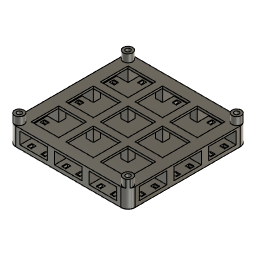
board_holder_outer_ziptie (Autodesk Fusion 360 design; units mm, degrees)
Autodesk Fusion 360 part; units mm, degrees
note: some values were not read from the file. Chosen so that the rebuilt part matches the saved one: which face or edge a step refers to.
sketch "Sketch1" plane through (0, 0, 0) normal (0, 0, 1) x (1, 0, 0)
  line L0 (-45.5, -45.5) -> (45.5, -45.5) construction
  line L1 (45.5, -45.5) -> (45.5, 45.5) construction
  line L2 (45.5, 45.5) -> (-45.5, 45.5) construction
  line L3 (-45.5, 45.5) -> (-45.5, -45.5) construction
  line L4 (-45.5, -45.5) -> (45.5, 45.5) construction
  line L5 (45.5, -45.5) -> (-45.5, 45.5) construction
  circle A0 centre (-45.5, 45.5) radius 1.95
  circle A1 centre (45.5, 45.5) radius 1.95
  circle A2 centre (-45.5, -45.5) radius 1.95
  circle A3 centre (45.5, -45.5) radius 1.95
  line L6 (-50, 50) -> (50, 50)
  line L7 (50, 50) -> (50, -50)
  line L8 (50, -50) -> (-50, -50)
  line L9 (-50, -50) -> (-50, 50)
  line L10 (-50, 50) -> (50, -50) construction
  line L11 (50, 50) -> (-50, -50) construction
  circle A4 centre (-45.5, 45.5) radius 3.95
  circle A5 centre (45.5, 45.5) radius 3.95
  circle A6 centre (-45.5, -45.5) radius 3.95
  circle A7 centre (45.5, -45.5) radius 3.95
  dimension "d1" = 91
  dimension "d2" = 91
  dimension "d3" = 3.9
  dimension "d6" = 91
  dimension "d8" = 100
  dimension "d9" = 7.9
  dimension "d12" = 91
  dimension "d102" = 100
  constraint perpendicular L0 L1
  constraint parallel L0 L2
  constraint parallel L1 L3
  constraint horizontal L0
  constraint coincident L4 origin
  constraint coincident L5 origin
  constraint coincident L2.end L3.start
  constraint perpendicular L6 L7
  constraint parallel L6 L8
  constraint parallel L7 L9
  constraint horizontal L6
  constraint coincident L10 origin
  constraint coincident L11 origin
  constraint concentric A0 A4
  measures "d1" distance of L1.end L2.end
  measures "d2" distance of L0.end L1.end
  measures "d3" diameter of A0
  measures "d8" distance of L7.end L8.end
  measures "d9" diameter of A4
  measures "d102" distance of L6.start L8.end
extrude "Extrude1" add sketch "Sketch1" along normal blind 18.5 contours A4 | A5 | A6 | A7 makes body 1 at (-41.5696, 45.1067, 6.1667) makes body 2 at (49.4304, 45.1067, 6.1667) makes body 3 at (-41.5696, -45.8933, 6.1667) makes body 4 at (49.4304, -45.8933, 6.1667)
extrude "Extrude2" add sketch "Sketch1" against normal blind 3.5 contours L6 L7 L8 L9 | A4 | A5 | A6 | A7 bodies 1 2 3 4
extrude "Extrude3" add sketch "Sketch1" along normal blind 12 contours L6 L7 L8 L9 bodies 1
sketch "Sketch2" plane through (0, -50, 0) normal (0, -1, 0) x (1, 0, 0)
  line L0 (50, -3.5) -> (50, 12)
  line L1 (-50, 12) -> (-40.5, 12)
  line L2 (-40.5, 12) -> (-40.5, -3.5)
  line L3 (-40.5, -3.5) -> (-50, -3.5)
  line L4 (-50, -3.5) -> (-50, 12)
  line L5 (-40.5, 12) -> (-17.5, 12)
  line L6 (-17.5, 12) -> (-17.5, -3.5)
  line L7 (-17.5, -3.5) -> (-40.5, -3.5)
  line L8 (-40.5, -3.5) -> (-40.5, 12)
  line L9 (-50, 12) -> (-50, 10)
  line L10 (-50, -3.5) -> (-50, 0)
  line L11 (-50, 10) -> (50, 10)
  line L12 (-50, 0) -> (50, 0)
  point P0 (-50, 12)
  dimension "d64" = 15.5
  dimension "d65" = 9.5
  dimension "d66" = 15.5
  dimension "d67" = 23
  dimension "d68" = 2
  dimension "d69" = 3.5
  constraint horizontal L1
  constraint vertical L2
  constraint horizontal L3
  constraint vertical L4
  constraint horizontal L5
  constraint vertical L6
  constraint horizontal L7
  constraint vertical L8
  constraint perpendicular L1 L9
  constraint perpendicular L3 L10
  constraint coincident L0 L11.end
  constraint perpendicular L0 L11
  constraint coincident L0 L12.end
  constraint perpendicular L0 L12
  constraint coincident P0 L1.start
  measures "d64" distance of P0 L3.end
  measures "d65" distance of P0 L1.end
  measures "d66" distance of L1.end L2.end
  measures "d67" distance of L1.end L5.end
  measures "d68" distance of P0 L9.end
  measures "d69" distance of L3.end L10.end
sketch "Sketch3" plane through (50, 0, 0) normal (1, 0, 0) x (0, 1, 0)
  line L0 (-50, 12) -> (-50, -3.5)
  line L1 (-50, -3.5) -> (50, -3.5)
  line L2 (50, -3.5) -> (50, 12)
  line L3 (50, 12) -> (-50, 12)
  line L4 (-50, 12) -> (-40.5, 12)
  line L5 (-40.5, 12) -> (-40.5, -3.5)
  line L6 (-40.5, -3.5) -> (-50, -3.5)
  line L7 (-50, -3.5) -> (-50, 12)
  line L8 (-40.5, 12) -> (-17.5, 12)
  line L9 (-17.5, 12) -> (-17.5, -3.5)
  line L10 (-17.5, -3.5) -> (-40.5, -3.5)
  line L11 (-40.5, -3.5) -> (-40.5, 12)
  line L12 (-50, 12) -> (-50, 10.3)
  line L13 (-50, -3.5) -> (-50, 0)
  line L14 (-50, 10.3) -> (50, 10.3)
  line L15 (-50, 0) -> (50, 0)
  dimension "d85" = 9.5
  dimension "d86" = 15.5
  dimension "d87" = 23
  dimension "d88" = 15.5
  dimension "d89" = 1.7
  dimension "d90" = 3.5
  constraint horizontal L4
  constraint vertical L5
  constraint horizontal L6
  constraint vertical L7
  constraint coincident L0.start L3.end
  constraint horizontal L8
  constraint vertical L9
  constraint horizontal L10
  constraint vertical L11
  constraint perpendicular L3 L12
  constraint coincident L0.end L1.start
  constraint perpendicular L6 L13
  constraint coincident L2 L14.end
  constraint perpendicular L2 L14
  constraint coincident L2 L15.end
  constraint perpendicular L2 L15
  measures "d85" distance of L0.start L4.end
  measures "d86" distance of L0.start L0.end
  measures "d87" distance of L4.end L8.end
  measures "d88" distance of L4.end L5.end
  measures "d89" distance of L0.start L12.end
  measures "d90" distance of L0.end L13.end
sketch "Sketch4" plane through (0, 0, -3.5) normal (0, 0, -1) x (1, 0, 0)
  circle A0 centre (-45.5, 45.5) radius 1.95
  circle A1 centre (45.5, 45.5) radius 1.95
  line L0 (50, 50) -> (-50, 50)
  line L1 (-50, 50) -> (-50, -50)
  line L2 (-50, -50) -> (50, -50)
  line L3 (50, -50) -> (50, 50)
  line L4 (45.5, 45.5) -> (18.5, 45.5)
  line L5 (18.5, 45.5) -> (18.5, 18.5)
  line L6 (18.5, 18.5) -> (45.5, 18.5)
  line L7 (45.5, 18.5) -> (45.5, 45.5)
  circle A2 centre (18.5, 18.5) radius 6.5
  circle A3 centre (-45.5, -45.5) radius 1.95
  circle A4 centre (45.5, -45.5) radius 1.95
  dimension "d43" = 27
  dimension "d44" = 27
  dimension "d45" = 13
  constraint horizontal L4
  constraint vertical L5
  constraint horizontal L6
  constraint vertical L7
  constraint coincident A1.centre L4.start
  constraint coincident L5.end L6.start
  measures "d43" distance of A1.centre L4.end
  measures "d44" distance of A1.centre L6.end
  measures "d45" diameter of A2
extrude "Extrude10" cut sketch "Sketch3" against normal blind 100 contours L5 L9 L11 L14 L15 bodies 1
pattern_linear "R-Pattern2" count 3 spacing 29 along (0, 1, 0) of "Extrude10"
extrude "Extrude9" cut sketch "Sketch2" against normal blind 100 contours L2 L6 L8 L11 L12 bodies 1
pattern_linear "R-Pattern1" count 3 spacing 29 along (1, 0, 0) of "Extrude9"
ref_plane "WorkPlane1" through (0, 0, 12) normal (0, 0, 1) x (1, 0, 0)
sketch "Sketch6" plane through (0, 0, 12) normal (0, 0, 1) x (1, 0, 0)
  line L0 (-50, 50) -> (50, 50) construction
  line L1 (50, 50) -> (50, -50) construction
  line L2 (50, -50) -> (-50, -50) construction
  line L3 (-50, -50) -> (-50, 50) construction
  line L4 (-50, 50) -> (50, -50) construction
  line L5 (50, 50) -> (-50, -50) construction
  line L6 (-50, -50) -> (-40.5, -50) construction
  line L7 (-40.5, -50) -> (-40.5, -40.5) construction
  line L8 (-40.5, -40.5) -> (-50, -40.5) construction
  line L9 (-50, -40.5) -> (-50, -50) construction
  line L10 (-40.5, -40.5) -> (-17.5, -40.5)
  line L11 (-17.5, -40.5) -> (-17.5, -17.5)
  line L12 (-17.5, -17.5) -> (-40.5, -17.5)
  line L13 (-40.5, -17.5) -> (-40.5, -40.5)
  dimension "d106" = 100
  dimension "d107" = 100
  dimension "d108" = 9.5
  dimension "d109" = 9.5
  dimension "d110" = 23
  dimension "d111" = 23
  constraint perpendicular L0 L1
  constraint parallel L0 L2
  constraint parallel L1 L3
  constraint horizontal L0
  constraint coincident L4 origin
  constraint coincident L5 origin
  constraint horizontal L6
  constraint vertical L7
  constraint horizontal L8
  constraint vertical L9
  constraint horizontal L10
  constraint vertical L11
  constraint horizontal L12
  constraint vertical L13
  measures "d106" distance of L1.end L2.end
  measures "d107" distance of L0.end L1.end
  measures "d108" distance of L2.end L6.end
  measures "d109" distance of L2.end L8.end
  measures "d110" distance of L7.end L10.end
  measures "d111" distance of L7.end L12.end
extrude "Extrude11" cut sketch "Sketch6" against normal blind 2 bodies 1
pattern_linear "R-Pattern3" count 3 spacing 29 along (0, 1, 0) count 3 spacing 29 along (1, 0, 0) of "Extrude11"
fillet "Fillet1" radius 6 4 edges at (-50, -50, 4.25) (50, -50, 4.25) (50, 50, 4.25) (-50, 50, 4.25) on bodies 1
chamfer "Chamfer3" distance 0.4 angle 45 12 edges at (-47.318, -46.2052, -3.5) (43.682, -46.2052, -3.5) (43.682, 44.7948, -3.5) (-47.318, 44.7948, -3.5) (0, 50, -3.5) (-48.2426, 48.2426, -3.5) (-50, 0, -3.5) (-48.2426, -48.2426, -3.5) (0, -50, -3.5) (48.2426, -48.2426, -3.5) (50, 0, -3.5) (48.2426, 48.2426, -3.5) on bodies 1
ref_plane "WorkPlane2" through (0, -46, 0) normal (0, 1, 0) x (0, 0, 1)
sketch "Sketch7" plane through (0, -46, 0) normal (0, 1, 0) x (1, 0, 0)
  line L0 (0, 0) -> (-50, 0) construction
  line L1 (-50, 0) -> (-40.5, 0) construction
  line L2 (-40.5, 0) -> (-29, 0) construction
  line L3 (-29, 0) -> (-29, 3.5) construction
  line L4 (-29, 0) -> (-27.625, 0) construction
  line L5 (-29, 0) -> (-33, 0) construction
  line L6 (-29, 3.5) -> (-40.5, 3.5) construction
  line L7 (-33, 0) -> (-33, 1)
  line L8 (-33, 0) -> (-35.5, 0)
  line L9 (-35.5, 0) -> (-35.5, 1)
  arc A0 (-33, 3.5) -> (-35.5, 1) centre (-33, 1) ccw
  line L10 (-33, 1) -> (-29, 1)
  line L11 (-33, 3.5) -> (-29, 3.5)
  line L12 (-29, 3.5) -> (-29, 1)
  arc A1 (-22.5, 1) -> (-25, 3.5) centre (-25, 1) ccw
  line L13 (-25, 0) -> (-22.5, 0)
  line L14 (-22.5, 0) -> (-22.5, 1)
  line L15 (-25, 0) -> (-25, 1)
  line L16 (-25, 1) -> (-29, 1)
  line L17 (-29, 3.5) -> (-17.5, 3.5) construction
  line L18 (-25, 3.5) -> (-29, 3.5)
  dimension "d121" = 50
  dimension "d122" = 9.5
  dimension "d123" = 11.5
  dimension "d124" = 3.5
  dimension "d126" = 4
  dimension "d127" = 11.5
  dimension "d128" = 1
  dimension "d129" = 2.5
  dimension "d130" = 1
  constraint coincident L0.start origin
  constraint horizontal L0
  constraint parallel L0 L1
  constraint parallel L0 L2
  constraint perpendicular L2 L3
  constraint perpendicular L3 L4
  constraint perpendicular L3 L5
  constraint perpendicular L3 L6
  constraint perpendicular L5 L7
  constraint perpendicular L7 L8
  constraint perpendicular L0 L9
  constraint coincident L6 A0.start
  constraint coincident L7.end A0.centre
  constraint coincident L3 L10.end
  constraint perpendicular L3 L10
  constraint symmetric L3.end L12 L6.start
  constraint symmetric L5.end L12 L13.start
  constraint symmetric L6.end L12 L17.end
  constraint symmetric L7.end L12 A1.centre
  constraint symmetric L8.end L12 L13.end
  constraint symmetric L9.end L12 A1.start
  constraint symmetric A0.start L12 A1.end
  constraint symmetric A0 L12 A1
  constraint symmetric L10.end L12 L16.end
  measures "d121" distance of L0.start L0.end
  measures "d122" distance of L0.end L1.end
  measures "d123" distance of L1.end L2.end
  measures "d124" distance of L2.end L3.end
  measures "d126" distance of L2.end L5.end
  measures "d127" distance of L3.end L6.end
  measures "d128" distance of L5.end L7.end
  measures "d129" distance of L5.end L8.end
  measures "d130" distance of L8.end L9.end
extrude "Extrude12" cut sketch "Sketch7" along normal blind 2 bodies 1
extrude "Extrude13" cut sketch "Sketch7" against normal blind 2 bodies 1
chamfer "Chamfer4" distance 1 distance2 1 2 edges at (-35.5, -46, 0) (-22.5, -46, 0) measured on face at (-30.3333, -26.3333, 0) measured on face at (-30.3333, -26.3333, 0) on bodies 1
fillet "Fillet2" radius 3 2 edges at (-35.5, -46, -0.9998) (-22.5, -46, -0.9998) on bodies 1
pattern_linear "R-Pattern4" count 3 spacing 29 along (1, 0, 0) count 2 spacing 92.5 along (0, 1, 0) of "Extrude12", "Extrude13", "Chamfer4", "Fillet2"
ref_plane "WorkPlane3" through (46, 0, 0) normal (1, 0, 0) x (0, 1, 0)
sketch "Sketch8" plane through (46, 0, 0) normal (1, 0, 0) x (0, 1, 0)
  line L0 (0, 0) -> (-50, 0) construction
  line L1 (-50, 0) -> (-40.5, 0) construction
  line L2 (-40.5, 0) -> (-29, 0) construction
  line L3 (-29, 0) -> (-29, -1)
  line L4 (-29, 0) -> (-33, 0) construction
  line L5 (-33, 0) -> (-35.5, 0)
  line L6 (-33, 0) -> (-33, -1)
  line L7 (-35.5, 0) -> (-35.5, -1)
  arc A0 (-35.5, -1) -> (-33, -3.5) centre (-33, -1) ccw
  line L8 (-33, -1) -> (-35.5, -1) construction
  line L9 (-33, -1) -> (-33, -3.5) construction
  line L10 (-33, -1) -> (-29, -1)
  line L11 (-29, 0) -> (-29, -3.5) construction
  line L12 (-29, -3.5) -> (-33, -3.5)
  line L13 (-29, -3.5) -> (-25, -3.5)
  arc A1 (-25, -3.5) -> (-22.5, -1) centre (-25, -1) ccw
  line L14 (-22.5, 0) -> (-22.5, -1)
  line L15 (-25, 0) -> (-22.5, 0)
  line L16 (-25, 0) -> (-25, -1)
  line L17 (-25, -1) -> (-29, -1)
  dimension "d143" = 50
  dimension "d144" = 9.5
  dimension "d145" = 11.5
  dimension "d146" = 1
  dimension "d147" = 4
  dimension "d148" = 2.5
  dimension "d149" = 1
  dimension "d150" = 1
  dimension "d151" = 90
  dimension "d152" = 3.5
  constraint coincident L0.start origin
  constraint horizontal L0
  constraint parallel L0 L1
  constraint parallel L0 L2
  constraint perpendicular L2 L3
  constraint perpendicular L3 L4
  constraint parallel L2 L5
  constraint perpendicular L0 L6
  constraint perpendicular L2 L7
  constraint coincident L6.end A0.centre
  constraint perpendicular L2 L11
  constraint symmetric L3.end L11 L10.end
  constraint symmetric L4.end L11 L15.start
  constraint symmetric L5.end L11 L14.start
  constraint symmetric L6.end L11 A1.centre
  constraint symmetric L7.end L11 A1.end
  constraint symmetric A0.end L11 L13.end
  constraint symmetric A0 L11 A1
  constraint symmetric L12.start L11 L13.start
  measures "d143" distance of L0.start L0.end
  measures "d144" distance of L0.end L1.end
  measures "d145" distance of L1.end L2.end
  measures "d146" distance of L2.end L3.end
  measures "d147" distance of L2.end L4.end
  measures "d148" distance of L4.end L5.end
  measures "d149" distance of L4.end L6.end
  measures "d150" distance of L5.end L7.end
  measures "d151" angle of L8 L9
  measures "d152" distance of L2.end L11.end
extrude "Extrude14" cut sketch "Sketch8" along normal blind 2 bodies 1
extrude "Extrude15" cut sketch "Sketch8" against normal blind 2 bodies 1
chamfer "Chamfer5" distance 1 distance2 1 2 edges at (46, -35.5, 0) (46, -22.5, 0) measured on face at (28.8333, -28.8333, 0) measured on face at (28.8333, -28.8333, 0) on bodies 1
fillet "Fillet3" radius 3 2 edges at (46, -35.5, -0.9998) (46, -22.5, -0.9998) on bodies 1
pattern_linear "R-Pattern5" count 3 spacing 29 along (0, 1, 0) count 2 spacing 92.5 along (-1, 0, 0) of "Extrude14", "Extrude15", "Chamfer5", "Fillet3"
sketch "Sketch9" plane through (0, 0, -3.5) normal (0, 0, -1) x (1, 0, 0)
  line L0 (-44.5, -4) -> (-48.5, -4)
  line L1 (-48.5, -4) -> (-48.5, 4)
  line L2 (-48.5, 4) -> (-44.5, 4)
  line L3 (-44.5, 4) -> (-44.5, -4)
  line L4 (48, -33) -> (44, -33)
  line L5 (44, -33) -> (44, -25)
  line L6 (44, -25) -> (48, -25)
  line L7 (48, -25) -> (48, -33)
  line L8 (48, 25) -> (44, 25)
  line L9 (44, 25) -> (44, 33)
  line L10 (44, 33) -> (48, 33)
  line L11 (48, 33) -> (48, 25)
  line L12 (-4, -48.5) -> (-4, -44.5)
  line L13 (-4, -44.5) -> (4, -44.5)
  line L14 (4, -44.5) -> (4, -48.5)
  line L15 (4, -48.5) -> (-4, -48.5)
  line L16 (25, 44) -> (25, 48)
  line L17 (25, 48) -> (33, 48)
  line L18 (33, 48) -> (33, 44)
  line L19 (33, 44) -> (25, 44)
  line L20 (-33, 44) -> (-33, 48)
  line L21 (-33, 48) -> (-25, 48)
  line L22 (-25, 48) -> (-25, 44)
  line L23 (-25, 44) -> (-33, 44)
  circle A0 centre (-45.5, -45.5) radius 2.35
  circle A1 centre (45.5, 45.5) radius 2.35
  circle A2 centre (-45.5, 45.5) radius 2.35
  circle A3 centre (45.5, -45.5) radius 2.35
  line L24 (-44, -49.6) -> (44, -49.6)
  arc A4 (44, -49.6) -> (49.6, -44) centre (44, -44) ccw
  line L25 (49.6, -44) -> (49.6, 44)
  arc A5 (49.6, 44) -> (44, 49.6) centre (44, 44) ccw
  line L26 (44, 49.6) -> (-44, 49.6)
  arc A6 (-44, 49.6) -> (-49.6, 44) centre (-44, 44) ccw
  line L27 (-49.6, 44) -> (-49.6, -44)
  arc A7 (-49.6, -44) -> (-44, -49.6) centre (-44, -44) ccw
  line L28 (-4, 44) -> (-4, 48)
  line L29 (-4, 48) -> (4, 48)
  line L30 (4, 48) -> (4, 44)
  line L31 (4, 44) -> (-4, 44)
  line L32 (-33, -48.5) -> (-33, -44.5)
  line L33 (-33, -44.5) -> (-25, -44.5)
  line L34 (-25, -44.5) -> (-25, -48.5)
  line L35 (-25, -48.5) -> (-33, -48.5)
  line L36 (25, -48.5) -> (25, -44.5)
  line L37 (25, -44.5) -> (33, -44.5)
  line L38 (33, -44.5) -> (33, -48.5)
  line L39 (33, -48.5) -> (25, -48.5)
  line L40 (48, -4) -> (44, -4)
  line L41 (44, -4) -> (44, 4)
  line L42 (44, 4) -> (48, 4)
  line L43 (48, 4) -> (48, -4)
  line L44 (-44.5, 25) -> (-48.5, 25)
  line L45 (-48.5, 25) -> (-48.5, 33)
  line L46 (-48.5, 33) -> (-44.5, 33)
  line L47 (-44.5, 33) -> (-44.5, 25)
  line L48 (-44.5, -33) -> (-48.5, -33)
  line L49 (-48.5, -33) -> (-48.5, -25)
  line L50 (-48.5, -25) -> (-44.5, -25)
  line L51 (-44.5, -25) -> (-44.5, -33)
  line L52 (45.5, 45.5) -> (18, 45.5) construction
  line L53 (18, 45.5) -> (18, 19.5) construction
  line L54 (18, 19.5) -> (45.5, 19.5) construction
  line L55 (45.5, 19.5) -> (45.5, 45.5) construction
  circle A8 centre (18, 19.5) radius 6.5
  dimension "d164" = 26
  dimension "d165" = 27.5
  dimension "d166" = 13
  constraint horizontal L52
  constraint vertical L53
  constraint horizontal L54
  constraint vertical L55
  constraint coincident A1.centre L52.start
  constraint coincident L53.end L54.start
  measures "d164" distance of A1.centre L54.end
  measures "d165" distance of A1.centre L52.end
  measures "d166" diameter of A8
extrude "Extrude17" [suppressed]
extrude "Extrude18" [suppressed]
extrude "Extrude16" [suppressed]
chamfer "Chamfer7" [suppressed]
delete_face "DeleteFace2" [suppressed]
chamfer "Chamfer8" [suppressed]
delete_face "DeleteFace3" [suppressed]
delete_face "DeleteFace4" [suppressed]
equation "d1 = PWidth"
equation "d2 = PLength"
equation "d3 = BoltClearence"
equation "d6 = PWidth"
equation "d7 = -PLength"
equation "d8 = BWidth"
equation "d9 = d3 + 4 mm"
equation "d12 = PWidth"
equation "d13 = -PLength"
equation "d14 = PegH"
equation "d16 = -Bottom"
equation "d18 = InnerHeight + XTop"
equation "BWidth = PWidth + 9 mm"
equation "Ends = 9.5 mm"
equation "InnerWalls = 6 mm"
equation "InnerHeight = 10 mm"
equation "XChamberW = ( ( BWidth - ( Ends * 2 ) - ( InnerWalls * ( XChannels - 1 ) ) ) / XChannels )"
equation "Bottom = 3.5 mm"
equation "XTop = 2 mm"
equation "XChamberH = Bottom + XTop + InnerHeight"
equation "PegH = 22 mm - Bottom"
equation "d64 = XChamberH"
equation "d65 = Ends"
equation "d66 = XChamberH"
equation "d67 = XChamberW"
equation "d68 = XTop"
equation "d69 = Bottom"
equation "XChannels = 3"
equation "d79 = -BLength"
equation "d81 = XChannels"
equation "d83 = -( XChamberW + InnerWalls ) * ( XChannels - 1 )"
equation "d85 = Ends"
equation "d86 = XChamberH"
equation "d87 = YChamberW"
equation "d88 = YChamberH"
equation "d89 = YTop"
equation "d90 = Bottom"
equation "d91 = -BWidth"
equation "d93 = YChannels"
equation "d95 = ( YChamberW + InnerWalls ) * ( YChannels - 1 )"
equation "BLength = PLength + 9 mm"
equation "YChamberW = ( ( BLength - ( Ends * 2 ) - ( InnerWalls * ( YChannels - 1 ) ) ) / YChannels )"
equation "YChamberH = Bottom + XTop + InnerHeight"
equation "YChannels = 3"
equation "d102 = BLength"
equation "PWidth = 91 mm"
equation "PLength = 91 mm"
equation "d105 = InnerHeight + XTop"
equation "d106 = BWidth"
equation "d107 = BLength"
equation "d108 = Ends"
equation "d109 = Ends"
equation "d110 = XChamberW"
equation "d111 = YChamberW"
equation "d112 = -XTop"
equation "d114 = YChannels"
equation "d115 = XChannels"
equation "d116 = ( YChamberW + InnerWalls ) * ( YChannels - 1 )"
equation "d117 = -( XChamberW + InnerWalls ) * ( XChannels - 1 )"
equation "d120 = ( -BLength / 2 ) + ( 4 mm )"
equation "d121 = BWidth / 2"
equation "d122 = Ends"
equation "d123 = XChamberW / 2"
equation "d124 = Bottom"
equation "d127 = XChamberW / 2"
equation "d138 = XChannels"
equation "d140 = ( XChamberW + InnerWalls ) * ( XChannels - 1 )"
equation "d141 = ( YChamberW + InnerWalls ) * ( YChannels ) + ( Ends - 4 mm )"
equation "d142 = ( BWidth / 2 ) - ( 4 mm )"
equation "d143 = BLength / 2"
equation "d144 = Ends"
equation "d145 = YChamberW / 2"
equation "d160 = YChannels"
equation "d162 = ( YChamberW + InnerWalls ) * ( YChannels - 1 )"
equation "d163 = ( XChamberW + InnerWalls ) * ( XChannels ) + ( Ends - 4 mm )"
equation "BoltClearence = 3.9 mm"
equation "YTop = XTop - 0.3 mm"
